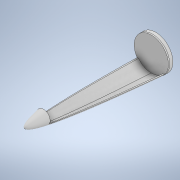
# Autodesk Inventor part: nose-basepart1
Saved by Autodesk Inventor 2020.3 (Build 243373000, 373)
## iProperties
Created: 2021-03-10
Part Number: nose-basepart1
Material: Generic
Document SubType Name: Modeling
Designer: 0x6f736f646f
Density: 1 g/cm^3
Appearance: Default
Author: 0x6f736f646f
Autodesk Inventor part; units mm, degrees
ref_plane "YZ Plane" through (0, 0, 0) normal (1, 0, 0) x (0, 1, 0)
ref_plane "XZ Plane" through (0, 0, 0) normal (0, 1, 0) x (-1, 0, 0)
ref_plane "XY Plane" through (0, 0, 0) normal (0, 0, 1) x (1, 0, 0)
sketch "Sketch2" plane through (0, 0, 0) normal (1, 0, 0) x (0, 1, 0)
  line L0 (0, 0) -> (25, 0)
  line L1 (25, 0) -> (25, -5)
  line L2 (25, -5) -> (26.8, -5)
  line L3 (26.8, -5) -> (26.8, 0)
  line L4 (0, 0) -> (-25, 0)
  line L5 (0, 0) -> (0, 200)
  line L6 (-25, 0) -> (-26.8, 0)
  spline S0 degree 2 poles (26.8, 0) (13.4, 200) (0, 200) knots 0 0 0 0.5 0.5 0.5
  line L7 (0, 0) -> (0, 198.2)
  spline S1 degree 2 poles (25, 0) (12.5, 198.2) (0, 198.2) knots 0 0 0 0.5 0.5 0.5
  line L8 (0, 2) -> (26.6657, 2)
  line L9 (0, 170) -> (0, 0)
  line L10 (0, 0) -> (0, 170)
  line L11 (0, 170) -> (10.3796, 170)
  line L12 (0, 172) -> (10.0276, 172)
  line L13 (1.8152, 198.2) -> (-1.8152, 198.2) construction
  arc A0 (1.0681, 197.7831) -> (-1.0681, 197.7831) centre (0, 196.6233) ccw construction
  line L14 (1.9566, 200) -> (-1.9566, 200) construction
  arc A1 (1.1799, 199.5579) -> (-1.1799, 199.5579) centre (0, 198.2044) ccw construction
  line L15 (0, 0) -> (-6, 0)
  line L16 (0, 170) -> (0, 0)
  line L17 (0, 2) -> (-5, 2)
  line L18 (-5, 2) -> (-5, 170)
  line L19 (-5, 170) -> (0, 170)
  line L20 (0, 170) -> (0, 2)
  line L21 (-5, 2) -> (-15, 2)
  line L22 (-15, 2) -> (-5, 170)
  point P0 (9.0895, 172)
  point P1 (0, 172)
  point P2 (0, 170)
  point P3 (9.43, 170)
  point P4 (24.8735, 2)
  point P5 (0, 170)
  dimension "d15" = 25
  dimension "d16" = 5
  dimension "d17" = 1.8
  dimension "d18" = 25
  dimension "d19" = 200
  dimension "d20" = 1.8
  dimension "d21" = 198.2
  dimension "d23" = 2
  dimension "d30" = 5
  dimension "d31" = 10
  constraints: 46 end point, 10 horizontal, 4 midpoint, 3 parallel, 3 perpendicular, 3 point on line, 2 centre point, 2 collinear, 2 point on circle, 2 vertical, 9 other
  measures "d15" distance of L0.start L0.end
  measures "d16" distance of L0.end L1.end
  measures "d17" distance of L1.end L2.end
  measures "d18" distance of L0.start L4.end
  measures "d19" distance of L5.end L0.start
  measures "d20" distance of L4.end L6.end
  measures "d21" distance of L7.end L0.start
  measures "d23" distance between parallel lines of L11 L12
  measures "d30" distance of L18.end L19.end
  measures "d31" distance of L17.end L21.end
revolve "Revolution3" add sketch "Sketch2" angle 360 mid plane about axis through (0, 0, 0) along (0, 0, 1) contours L5 L8 S1 L0 | S1 L8 S0 L3 L2 L1 | S1 L11 S0 L8 | L5 L12 S1 L11 | S1 L12 S0 L11 | S1 L5 S0 L12
extrude "Extrusion2" cut sketch "Sketch2" against normal mid plane 60 contours L17 L18 L19 L5 | L5 L11 S1 L8 | S1 L11 S0 L8 | L21 L22 L18
body "Solid2"
